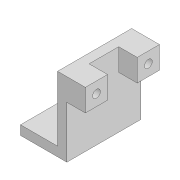
# Autodesk Inventor part: suporte_termopar
Saved by Autodesk Inventor 2020 (Build 240168000, 168)
## iProperties
Created: 2022-07-21
Part Number: suporte_termopar
Material: Genérico
Document SubType Name: Modeling
Designer: gabri
Density: 1 g/cm^3
Appearance: Padrão
Author: gabri
Autodesk Inventor part; units mm, degrees
ref_plane "YZ Plane" through (0, 0, 0) normal (1, 0, 0) x (0, 1, 0)
ref_plane "XZ Plane" through (0, 0, 0) normal (0, 1, 0) x (-1, 0, 0)
ref_plane "XY Plane" through (0, 0, 0) normal (0, 0, 1) x (1, 0, 0)
sketch "Esboço1" plane through (0, 0, 0) normal (0, 0, 1) x (1, 0, 0)
  line L0 (0, 0) -> (25, 0)
  line L1 (25, 0) -> (25, 40)
  line L2 (25, 40) -> (0, 40)
  line L3 (0, 40) -> (0, 0)
  dimension "d0" = 25
  dimension "d1" = 40
  constraints: 8 end point, 2 parallel, 1 horizontal, 1 perpendicular
  measures "d0" distance of L1.end L2.end
  measures "d1" distance of L2.end L0.start
extrude "Extrusão1" add sketch "Esboço1" along normal blind 40
sketch "Esboço2" plane through (0, 0, 0) normal (0, 0, -1) x (-1, 0, 0)
  line L0 (-25, 40) -> (0, 40) projected
  line L1 (0, 40) -> (-20, 40)
  line L2 (-20, 40) -> (-20, 5)
  line L3 (-20, 5) -> (0, 5)
  line L4 (0, 5) -> (0, 40)
  line L5 (-25, 0) -> (-25, 40) projected
  line L6 (0, 0) -> (-25, 0) projected
  dimension "d4" = 5
  dimension "d5" = 5
  constraints: 8 end point, 2 parallel, 1 horizontal, 1 perpendicular
  measures "d4" distance between parallel lines of L5 L2
  measures "d5" distance between parallel lines of L6 L3
extrude "Extrusão2" cut sketch "Esboço2" against normal blind 40
sketch "Esboço3" plane through (25, 0, 0) normal (1, 0, 0) x (0, 0, -1)
  line L0 (0, 40) -> (-12, 40)
  line L1 (-12, 40) -> (-12, 28)
  line L2 (-12, 28) -> (0, 28)
  line L3 (0, 28) -> (0, 40)
  line L4 (-40, 40) -> (-28, 40)
  line L5 (-28, 40) -> (-28, 28)
  line L6 (-28, 28) -> (-40, 28)
  line L7 (-40, 28) -> (-40, 40)
  line L8 (0, 40) -> (-40, 40) projected
  line L9 (-40, 0) -> (-40, 40) projected
  circle A0 centre (-6, 34) radius 2.1
  circle A1 centre (-34, 34) radius 2.1
  point P0 (0, 0)
  dimension "d8" = 12
  dimension "d9" = 0
  dimension "d10" = 0
  dimension "d11" = 12
  dimension "d12" = 12
  dimension "d13" = 4.2
  dimension "d14" = 4.2
  dimension "d17" = 6
  dimension "d18" = 6
  dimension "d19" = 6
  dimension "d20" = 6
  constraints: 16 end point, 4 parallel, 2 centre point, 2 horizontal, 2 perpendicular, 2 point on line
  measures "d8" distance of L2.end L0.start
  measures "d9" distance between parallel lines of L8 L0
  measures "d10" distance between parallel lines of L9 L7
  measures "d11" distance of L1.end L2.end
  measures "d12" distance of L5.end L6.end
  measures "d13" diameter of A0
  measures "d14" diameter of A1
  measures "d17" distance from line of L3 A0.centre
  measures "d18" distance from line of L2 A0.centre
  measures "d19" distance from line of A1.centre L6
  measures "d20" distance from line of L5 A1.centre
extrude "Extrusão3" add sketch "Esboço3" along normal blind 10
sketch "Esboço4" plane through (35, 0, 0) normal (1, 0, 0) x (0, 0, -1)
  circle A0 centre (-6, 34) radius 2.1 projected
  circle A1 centre (-34, 34) radius 2.1 projected
  point P0 (0, 0)
extrude "Extrusão4" cut sketch "Esboço4" against normal blind 50
sketch "Esboço5" plane through (20, 5, 0) normal (-1, 0, 0) x (0, 0, 1)
  circle A0 centre (34, 29) radius 2.1 projected
  circle A1 centre (6, 29) radius 2.1 projected
  line L0 (30.0163, 29) -> (32.0081, 32.45)
  line L1 (32.0081, 32.45) -> (35.9919, 32.45)
  line L2 (35.9919, 32.45) -> (37.9837, 29)
  line L3 (37.9837, 29) -> (35.9919, 25.55)
  line L4 (35.9919, 25.55) -> (32.0081, 25.55)
  line L5 (32.0081, 25.55) -> (30.0163, 29)
  line L6 (9.9837, 29) -> (7.9919, 25.55)
  line L7 (7.9919, 25.55) -> (4.0081, 25.55)
  line L8 (4.0081, 25.55) -> (2.0163, 29)
  line L9 (2.0163, 29) -> (4.0081, 32.45)
  line L10 (4.0081, 32.45) -> (7.9919, 32.45)
  line L11 (7.9919, 32.45) -> (9.9837, 29)
  line L12 (0, 35) -> (40, 35) projected
  point P0 (0, -5)
  dimension "d23" = 6.9
  dimension "d24" = 6.9
  constraints: 24 end point, 2 coincident, 2 parallel, 26 other
  measures "d23" distance between parallel lines of L0 L3
  measures "d24" distance between parallel lines of L10 L7
extrude "Extrusão5" cut sketch "Esboço5" against normal blind 6 contours A0 | A1 | L0 L1 L2 L3 L4 L5 | L6 L7 L8 L9 L10 L11
equation "\"d12\" = d11"
equation "\"d13\" = d14"
equation "\"d17\" = 0.5 * d11"
equation "\"d18\" = 0.5 * d8"
equation "\"d19\" = d18"
equation "\"d20\" = d17"
equation "\"d24\" = d23"
